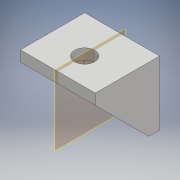
# Autodesk Inventor part: Gabarito Furo BOX
Saved by Autodesk Inventor 2017 (Build 210142000, 142)
## iProperties
Created: 2020-07-30
Part Number: Gabarito Furo BOX
Material: Generic
Document SubType Name: Modeling
Designer: ale
Density: 1 g/cm^3
Appearance: Default
Author: ale
Autodesk Inventor part; units mm, degrees
ref_plane "YZ Plane" through (0, 0, 0) normal (1, 0, 0) x (0, 1, 0)
ref_plane "XZ Plane" through (0, 0, 0) normal (0, 1, 0) x (-1, 0, 0)
ref_plane "XY Plane" through (0, 0, 0) normal (0, 0, 1) x (1, 0, 0)
sketch "Sketch1" plane through (0, 0, 0) normal (0, 0, 1) x (1, 0, 0)
  circle A0 centre (0, 0) radius 3.75
  line L0 (-10, 10) -> (10, 10)
  line L1 (10, 10) -> (10, -10)
  line L2 (10, -10) -> (-10, -10)
  line L3 (-10, -10) -> (-10, 10)
  line L4 (-10, 10) -> (10, -10) construction
  line L5 (10, 10) -> (-10, -10) construction
  dimension "d0" = 7.5
  dimension "d1" = 20
  dimension "d2" = 20
  constraints: 12 end point, 2 midpoint, 2 parallel, 1 centre point, 1 coincident, 1 horizontal, 1 perpendicular
  measures "d0" diameter of A0
  measures "d1" distance of L0.end L1.end
  measures "d2" distance between parallel lines of L1 L3
extrude "Extrusion1" add sketch "Sketch1" along normal blind 4
sketch "Sketch2" plane through (-10, 10, 0) normal (0, 1, 0) x (1, 0, 0)
  line L0 (20, -4) -> (0, -4) projected
  line L1 (0, -4) -> (20, -4)
  line L2 (20, -4) -> (20, 20)
  line L3 (20, 20) -> (0, 20)
  line L4 (0, 20) -> (0, -4)
  point P0 (10, 0)
  dimension "d5" = 24
  constraints: 8 end point, 2 parallel, 1 horizontal, 1 perpendicular
  measures "d5" distance of L2.end L1.end
extrude "Extrusion2" add sketch "Sketch2" along normal blind 4
sketch "Sketch3" plane through (10, -10, 4) normal (1, 0, 0) x (0, 0, -1)
  line L0 (4, 0) -> (0, 0) projected
  line L1 (4, 20) -> (24, 20) projected
  line L2 (4, 0) -> (24, 20)
  line L3 (24, 20) -> (24, 24) projected
  line L4 (24, 20) -> (24, 24)
  line L5 (24, 24) -> (0, 24) projected
  line L6 (24, 24) -> (0, 24)
  line L7 (0, 0) -> (0, 24) projected
  line L8 (0, 24) -> (0, 0)
  line L9 (0, 0) -> (4, 0)
  point P0 (4, 10)
  constraints: 10 end point, 3 collinear, 1 perpendicular
extrude "Extrusion3" add sketch "Sketch3" along normal blind 4
ref_plane "Work Plane1" through (0, -10, 4) normal (1, 0, 0) x (0, 0, -1)
mirror "Mirror1" about plane through (0, -10, 4) normal (1, 0, 0) of "Extrusion3"
sketch "Sketch4" plane through (14, 10, -20) normal (0, 0, -1) x (-1, 0, 0)
  line L0 (3.5, 0) -> (24.5, 0)
  line L1 (24.5, 0) -> (24.5, -20)
  line L2 (24.5, -20) -> (3.5, -20)
  line L3 (3.5, -20) -> (3.5, 0)
  line L4 (3.5, 0) -> (24.5, -20) construction
  line L5 (24.5, 0) -> (3.5, -20) construction
  point P0 (14, -10)
  dimension "d11" = 21
  dimension "d12" = 20
  constraints: 12 end point, 2 midpoint, 2 parallel, 1 horizontal, 1 perpendicular
  measures "d11" distance of L1.end L2.end
  measures "d12" distance of L0.end L1.end
extrude "Extrusion4" cut sketch "Sketch4" against normal blind 20
body "Solid1"
